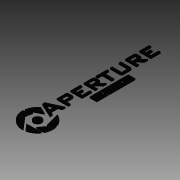
# Autodesk Inventor part: logo_full
Saved by Autodesk Inventor 2015 (Build 190159000, 159)
## iProperties
Created: 2014-10-14
Part Number: logo_full
Material: Generic
Document SubType Name: Modeling
Designer: Adam
Density: 1 g/cm^3
Appearance: Black
Author: Adam
Autodesk Inventor part; units mm, degrees
ref_plane "YZ Plane" through (0, 0, 0) normal (1, 0, 0) x (0, 1, 0)
ref_plane "XZ Plane" through (0, 0, 0) normal (0, 1, 0) x (-1, 0, 0)
ref_plane "XY Plane" through (0, 0, 0) normal (0, 0, 1) x (1, 0, 0)
sketch "Sketch1" plane through (0, 0, 0) normal (0, 1, 0) x (-1, 0, 0)
  line L0 (50, 0) -> (50, -199.1582) construction
  line L1 (50, -199.1582) -> (0, -199.1582) construction
  line L2 (0, -199.1582) -> (0, 0) construction
  line L3 (0, 0) -> (50, 0) construction
  line L4 (60, 0) -> (-10, 0) projected
  arc A0 (5.1979, -32.7466) -> (17.2152, -44.0591) centre (25, -23.75) ccw
  line L5 (11.7, -24) -> (5.1979, -32.7466)
  line L6 (11.7, -24) -> (17.2152, -44.0591)
  circle A1 centre (25, -23.75) radius 5.75
  arc A2 (5.6494, -13.8195) -> (4.2484, -30.2641) centre (25, -23.75) ccw
  line L7 (16.5428, -13.4822) -> (5.6494, -13.8195)
  line L8 (16.5428, -13.4822) -> (4.2484, -30.2641)
  arc A3 (20.7629, -2.4167) -> (7.0051, -11.5333) centre (25, -23.75) ccw
  line L9 (27.7937, -10.7443) -> (20.7629, -2.4167)
  line L10 (27.7937, -10.7443) -> (7.0051, -11.5333)
  arc A4 (39.0869, -7.1783) -> (23.3967, -2.0592) centre (25, -23.75) ccw
  line L11 (36.9278, -17.8609) -> (39.0869, -7.1783)
  line L12 (36.9278, -17.8609) -> (23.3967, -2.0592)
  arc A5 (46.7372, -24.4963) -> (41.0031, -9.0203) centre (25, -23.75) ccw
  line L13 (37.0241, -29.4397) -> (46.7372, -24.4963)
  line L14 (37.0241, -29.4397) -> (41.0031, -9.0203)
  arc A6 (37.9171, -41.2489) -> (46.4838, -27.1422) centre (25, -23.75) ccw
  line L15 (28.0098, -36.7074) -> (37.9171, -41.2489)
  line L16 (28.0098, -36.7074) -> (46.4838, -27.1422)
  line L17 (20.7257, -37.1631) -> (41.0031, -46.4582)
  line L18 (41.0031, -46.4582) -> (41.0031, -49.9857)
  line L19 (41.0031, -49.9857) -> (20.7257, -59.2364)
  line L20 (20.7257, -59.2364) -> (20.7257, -54.8042)
  line L21 (20.7257, -54.8042) -> (25.3171, -52.9285)
  line L22 (25.3171, -52.9285) -> (25.3171, -43.0274)
  line L23 (25.3171, -43.0274) -> (20.7257, -40.9227)
  line L24 (20.7257, -40.9227) -> (20.7257, -37.1631)
  line L25 (28.8648, -44.6536) -> (36.7381, -48.2627)
  line L26 (36.7381, -48.2627) -> (28.8648, -51.4791)
  line L27 (28.8648, -51.4791) -> (28.8648, -44.6536)
  line L28 (37.2257, -63.1991) -> (20.7257, -63.1991)
  line L29 (20.7257, -63.1991) -> (20.7257, -66.398)
  line L30 (27.2257, -66.398) -> (27.2257, -75.6295)
  line L31 (29.9757, -74.1295) -> (29.9757, -66.398)
  line L32 (37.2257, -63.1991) -> (37.2257, -75.6295)
  line L33 (34.4757, -74.1295) -> (34.4757, -66.398)
  arc A7 (34.7257, -78.1295) -> (37.2257, -75.6295) centre (34.7257, -75.6295) ccw
  arc A8 (27.2257, -75.6295) -> (29.7257, -78.1295) centre (29.7257, -75.6295) ccw
  line L34 (34.7257, -78.1295) -> (29.7257, -78.1295)
  line L35 (37.2257, -82.598) -> (20.7257, -82.598)
  line L36 (34.2257, -85.748) -> (34.2257, -96.6526)
  line L37 (34.2257, -96.6526) -> (37.2257, -96.6526)
  line L38 (37.2257, -96.6526) -> (37.2257, -82.598)
  line L39 (23.7257, -85.748) -> (23.7257, -96.6526)
  line L40 (23.7257, -96.6526) -> (20.7257, -96.6526)
  line L41 (20.7257, -96.6526) -> (20.7257, -82.598)
  arc A9 (33.4757, -75.1295) -> (34.4757, -74.1295) centre (33.4757, -74.1295) ccw
  arc A10 (29.9757, -74.1295) -> (30.9757, -75.1295) centre (30.9757, -74.1295) ccw
  line L42 (33.4757, -75.1295) -> (30.9757, -75.1295)
  line L43 (20.7257, -66.398) -> (27.2257, -66.398)
  line L44 (29.9757, -66.398) -> (34.4757, -66.398)
  line L45 (27.771, -85.748) -> (27.771, -92.1807)
  line L46 (27.771, -92.1807) -> (30.771, -92.1807)
  line L47 (30.771, -92.1807) -> (30.771, -85.748)
  line L48 (23.7257, -85.748) -> (27.771, -85.748)
  line L49 (30.771, -85.748) -> (34.2257, -85.748)
  line L50 (37.2257, -101.4125) -> (20.7257, -101.4125)
  line L51 (20.7257, -101.4125) -> (20.7257, -104.5625)
  arc A11 (33.4757, -113.1783) -> (34.4757, -112.1783) centre (33.4757, -112.1783) ccw
  arc A12 (29.9757, -112.1783) -> (30.9757, -113.1783) centre (30.9757, -112.1783) ccw
  line L52 (33.4757, -113.1783) -> (30.9757, -113.1783)
  line L53 (34.4757, -104.5625) -> (29.9757, -104.5625)
  line L54 (29.9757, -104.5625) -> (29.9757, -112.1783)
  line L55 (34.4757, -112.1783) -> (34.4757, -104.5625)
  arc A13 (34.7257, -116.1783) -> (37.2257, -113.6783) centre (34.7257, -113.6783) ccw
  arc A14 (27.2257, -113.6783) -> (29.7257, -116.1783) centre (29.7257, -113.6783) ccw
  line L56 (34.7257, -116.1783) -> (29.7257, -116.1783)
  line L57 (37.2257, -101.4125) -> (37.2257, -113.6783)
  line L58 (20.7257, -104.5625) -> (27.2257, -104.5625)
  line L59 (29.9757, -104.5625) -> (34.4757, -104.5625)
  line L60 (27.2257, -107.3837) -> (20.7257, -112.8855)
  line L61 (20.7257, -112.8855) -> (20.7257, -117.6583)
  line L62 (27.2257, -111.29) -> (20.7013, -117.6821)
  line L63 (37.2257, -101.4928) -> (37.2257, -101.4125)
  line L64 (37.2257, -113.6783) -> (37.2257, -113.1783)
  line L65 (37.2257, -101.4928) -> (37.2257, -101.4125)
  line L66 (37.2257, -118.6046) -> (34.2257, -118.6046)
  line L67 (34.2257, -134.6046) -> (37.2257, -134.6046)
  line L68 (37.2257, -134.6046) -> (37.2257, -118.6046)
  line L69 (34.2257, -124.8546) -> (20.7257, -124.8546)
  line L70 (20.7257, -124.8546) -> (20.7257, -128.3546)
  line L71 (20.7257, -128.3546) -> (34.2257, -128.3546)
  line L72 (34.2257, -118.6046) -> (34.2257, -124.8546)
  line L73 (34.2257, -128.3546) -> (34.2257, -134.6046)
  line L74 (37.2257, -126.6046) -> (20.7257, -126.6046) construction
  line L75 (27.2257, -104.5625) -> (27.2257, -107.3837)
  line L76 (27.2257, -111.29) -> (27.2257, -113.6783)
  line L77 (37.2257, -160.0956) -> (20.7257, -160.0956)
  line L78 (20.7257, -160.0956) -> (20.7257, -163.2456)
  arc A15 (33.4684, -171.8614) -> (34.4684, -170.8614) centre (33.4684, -170.8614) ccw
  arc A16 (29.9684, -170.8614) -> (30.9684, -171.8614) centre (30.9684, -170.8614) ccw
  line L79 (33.4684, -171.8614) -> (30.9684, -171.8614)
  line L80 (34.4684, -163.2456) -> (29.9684, -163.2456)
  line L81 (29.9684, -163.2456) -> (29.9684, -170.8614)
  line L82 (34.4684, -170.8614) -> (34.4684, -163.2456)
  arc A17 (34.7257, -174.8614) -> (37.2257, -172.3614) centre (34.7257, -172.3614) ccw
  arc A18 (27.2184, -172.3614) -> (29.7184, -174.8614) centre (29.7184, -172.3614) ccw
  line L83 (34.7257, -174.8614) -> (29.7184, -174.8614)
  line L84 (37.2257, -160.0956) -> (37.2257, -172.3614)
  line L85 (20.7257, -163.2456) -> (27.2184, -163.2456)
  line L86 (29.9684, -163.2456) -> (34.4684, -163.2456)
  line L87 (27.2184, -166.0668) -> (20.7257, -171.5759)
  line L88 (20.7257, -171.5759) -> (20.7257, -176.3487)
  line L89 (27.2184, -169.9731) -> (20.7137, -176.3605)
  line L90 (37.2257, -160.1464) -> (37.2257, -160.0956)
  line L91 (37.2257, -172.3614) -> (37.2257, -171.8614)
  line L92 (37.2257, -160.1464) -> (37.2257, -160.0956)
  line L93 (27.2184, -163.2456) -> (27.2184, -166.0668)
  line L94 (27.2184, -169.9731) -> (27.2184, -172.3614)
  line L95 (37.2257, -180.2989) -> (20.7257, -180.2989)
  line L96 (34.2257, -183.4489) -> (34.2257, -194.3535)
  line L97 (34.2257, -194.3535) -> (37.2257, -194.3535)
  line L98 (37.2257, -194.3535) -> (37.2257, -180.2989)
  line L99 (23.7257, -183.4489) -> (23.7257, -194.3535)
  line L100 (23.7257, -194.3535) -> (20.7257, -194.3535)
  line L101 (20.7257, -194.3535) -> (20.7257, -180.2989)
  line L102 (27.771, -183.4489) -> (27.771, -189.8816)
  line L103 (27.771, -189.8816) -> (30.771, -189.8816)
  line L104 (30.771, -189.8816) -> (30.771, -183.4489)
  line L105 (23.7257, -183.4489) -> (27.771, -183.4489)
  line L106 (30.771, -183.4489) -> (34.2257, -183.4489)
  line L107 (37.2257, -138.6629) -> (23.4227, -138.6629)
  line L108 (23.7257, -141.8629) -> (37.2257, -141.8629)
  line L109 (37.2257, -141.8629) -> (37.2257, -138.6629)
  line L110 (37.2257, -150.938) -> (23.7257, -150.938)
  line L111 (23.4227, -154.138) -> (37.2257, -154.138)
  line L112 (37.2257, -154.138) -> (37.2257, -150.938)
  line L113 (23.7257, -150.938) -> (23.7257, -141.8629)
  arc A19 (20.7257, -151.4409) -> (23.4227, -154.138) centre (23.4227, -151.4409) ccw
  arc A20 (23.4227, -138.6629) -> (20.7257, -141.36) centre (23.4227, -141.36) ccw
  line L114 (20.7257, -141.36) -> (20.7257, -151.4409)
  line L115 (16.0446, -88.9644) -> (6.0602, -88.9644)
  line L116 (6.0602, -88.9644) -> (6.0602, -143.5469)
  line L117 (6.0602, -143.5469) -> (16.0446, -143.5469)
  line L118 (16.0446, -143.5469) -> (16.0446, -88.9644)
  dimension "d9" = 50
  dimension "d17" = 52
  dimension "d24" = 20.8035
  dimension "d25" = 21.75
  dimension "d26" = 11.7
  dimension "d28" = 24
  dimension "d54" = 25
  dimension "d56" = 23.75
  dimension "d57" = 11.5
  dimension "d64" = 258
  dimension "d252" = 2.5
  dimension "d255" = 16.5
  dimension "d258" = 6.5
  dimension "d259" = 2.75
  dimension "d260" = 2.75
  dimension "d261" = 1
  dimension "d262" = 3.15
  dimension "d265" = 16.2
  dimension "d271" = 3
  dimension "d273" = 3
  dimension "d280" = 3
  dimension "d282" = 3
  dimension "d283" = 3
  dimension "d284" = 3.15
  dimension "d295" = 3
  dimension "d296" = 3.5
  dimension "d297" = 16
  dimension "d305" = 3
  dimension "d306" = 3.15
  dimension "d312" = 2.75
  dimension "d313" = 2.8212
  dimension "d320" = 16.5
  dimension "d321" = 3.15
  dimension "d322" = 3
  dimension "d323" = 3
  dimension "d324" = 3
  dimension "d351" = 3.2
  dimension "d352" = 3.2
  dimension "d353" = 3
  constraints: 228 end point, 45 parallel, 40 point on circle, 32 collinear, 30 tangent, 21 centre point, 16 horizontal, 10 point on line, 10 vertical, 9 perpendicular, 7 equal radius, 3 coincident, 2 midpoint, 1 vertical alignment, 37 other
  measures "d9" distance of L0.end L1.end
  measures "d17" angle of L5 L6
  measures "d24" distance of L5.start L6.end
  measures "d25" radius of A0
  measures "d26" distance from line of L2 L5.start
  measures "d28" distance from line of L3 L5.start
  measures "d54" distance from line of L2 A1.centre
  measures "d56" distance from line of L3 A1.centre
  measures "d57" diameter of A1
  measures "d252" radius of A7
  measures "d255" distance of L35.start L35.end
  measures "d258" distance between parallel lines of L41 L30
  measures "d259" distance between parallel lines of L31 L30
  measures "d260" distance between parallel lines of L32 L33
  measures "d261" radius of A9
  measures "d262" distance between parallel lines of L35 L49
  measures "d265" distance between parallel lines of L43 L35
  measures "d271" distance between parallel lines of L34 L42
  measures "d273" distance between parallel lines of L56 L52
  measures "d280" distance between parallel lines of L36 L38
  measures "d282" distance between parallel lines of L45 L47
  measures "d283" distance between parallel lines of L41 L39
  measures "d284" distance between parallel lines of L50 L53
  measures "d295" distance between parallel lines of L72 L68
  measures "d296" distance between parallel lines of L71 L69
  measures "d297" distance of L67.end L66.start
  measures "d305" distance between parallel lines of L83 L79
  measures "d306" distance between parallel lines of L77 L80
  measures "d312" distance between parallel lines of L81 L93
  measures "d313" distance of L93.start L93.end
  measures "d320" distance of L95.start L95.end
  measures "d321" distance between parallel lines of L95 L106
  measures "d322" distance between parallel lines of L96 L98
  measures "d323" distance between parallel lines of L102 L104
  measures "d324" distance between parallel lines of L101 L99
  measures "d351" distance of L111.end L110.start
  measures "d352" distance of L108.end L107.start
  measures "d353" distance between parallel lines of L114 L113
extrude "Extrusion1" add sketch "Sketch1" along normal blind 2
sketch "Sketch2" plane through (0, 2, 0) normal (0, 1, 0) x (1, 0, 0)
  line L0 (-14.0025, 91.7025) -> (-14.0025, 151.1401) construction
  line L1 (-14.0025, 151.1401) -> (-8.0025, 151.1401) construction
  line L2 (-8.0025, 151.1401) -> (-8.0025, 91.7025) construction
  line L3 (-8.0025, 91.7025) -> (-14.0025, 91.7025) construction
  line L4 (-8.0025, 126.4644) -> (-14.0025, 126.4644)
  line L5 (-14.0025, 126.4644) -> (-14.0025, 127.5644)
  line L6 (-14.0025, 127.5644) -> (-10.7116, 129.4644)
  line L7 (-10.7116, 129.4644) -> (-14.0025, 131.3644)
  line L8 (-14.0025, 131.3644) -> (-14.0025, 132.4644)
  line L9 (-14.0025, 132.4644) -> (-8.0025, 132.4644)
  line L10 (-8.0025, 132.4644) -> (-8.0025, 131.3644)
  line L11 (-8.0025, 131.3644) -> (-12.0025, 131.3644)
  line L12 (-12.0025, 131.3644) -> (-8.7116, 129.4644)
  line L13 (-8.7116, 129.4644) -> (-12.0025, 127.5644)
  line L14 (-12.0025, 127.5644) -> (-8.0025, 127.5644)
  line L15 (-8.0025, 126.4644) -> (-8.0025, 127.5644)
  line L16 (-6.0602, 88.9644) -> (-6.0602, 143.5469) projected
  line L17 (-16.0446, 88.9644) -> (-6.0602, 88.9644) projected
  line L18 (-12.7651, 96.9555) -> (-12.7651, 94.1247)
  line L19 (-12.7651, 94.1247) -> (-11.7554, 94.1247)
  line L20 (-11.7554, 94.1247) -> (-11.7554, 96.9263)
  spline S0 degree 2 poles (-11.7554, 96.9263) (-11.7554, 97.6675) (-11.1017, 98.2103) (-10.2788, 98.2103) knots 0 0 0 1 2 2 2
  line L21 (-10.2788, 98.2103) -> (-9.485, 98.2103)
  spline S1 degree 2 poles (-9.485, 98.2103) (-8.6562, 98.2103) (-8.0025, 97.6675) (-8.0025, 96.9263) knots 0 0 0 1 2 2 2
  line L22 (-8.0025, 96.9263) -> (-8.0025, 94.0372)
  spline S2 degree 2 poles (-8.0025, 94.0372) (-8.0025, 93.2901) (-8.6504, 92.7473) (-9.485, 92.7473) knots 0 0 0 1 2 2 2
  line L23 (-9.485, 92.7473) -> (-9.7243, 92.7473)
  line L24 (-9.7243, 92.7473) -> (-10.0044, 93.9438)
  line L25 (-10.0044, 93.9438) -> (-9.3157, 93.9438)
  line L26 (-9.3157, 93.9438) -> (-9.3157, 97.0138)
  line L27 (-9.3157, 97.0138) -> (-10.4072, 97.0138)
  line L28 (-10.4072, 97.0138) -> (-10.4072, 94.2181)
  spline S3 degree 2 poles (-10.4072, 94.2181) (-10.4072, 93.4769) (-11.0609, 92.9399) (-11.8897, 92.9399) knots 0 0 0 1 2 2 2
  line L29 (-11.8897, 92.9399) -> (-12.5258, 92.9399)
  spline S4 degree 2 poles (-12.5258, 92.9399) (-13.3546, 92.9399) (-14.0025, 93.4769) (-14.0025, 94.2181) knots 0 0 0 1 2 2 2
  line L30 (-14.0025, 94.2181) -> (-14.0025, 96.8737)
  spline S5 degree 2 poles (-14.0025, 96.8737) (-14.0025, 97.5858) (-13.3721, 98.1519) (-12.6251, 98.1519) knots 0 0 0 1 2 2 2
  line L31 (-12.6251, 98.1519) -> (-12.4149, 98.1519)
  line L32 (-12.4149, 98.1519) -> (-12.1114, 96.9555)
  line L33 (-12.1114, 96.9555) -> (-12.7651, 96.9555)
  line L34 (-8.0025, 101.6889) -> (-10.664, 101.6889)
  line L35 (-10.664, 101.6889) -> (-14.0025, 99.2609)
  line L36 (-14.0025, 99.2609) -> (-14.0025, 100.8893)
  line L37 (-14.0025, 100.8893) -> (-11.7904, 102.436)
  line L38 (-11.7904, 102.436) -> (-14.0025, 103.9827)
  line L39 (-14.0025, 103.9827) -> (-14.0025, 105.4418)
  line L40 (-14.0025, 105.4418) -> (-10.699, 103.0197)
  line L41 (-10.699, 103.0197) -> (-8.0025, 103.0197)
  line L42 (-8.0025, 103.0197) -> (-8.0025, 101.6889)
  line L43 (-12.7651, 110.6597) -> (-12.7651, 107.829)
  line L44 (-12.7651, 107.829) -> (-11.7554, 107.829)
  line L45 (-11.7554, 107.829) -> (-11.7554, 110.6305)
  spline S6 degree 2 poles (-11.7554, 110.6305) (-11.7554, 111.3718) (-11.1017, 111.9146) (-10.2788, 111.9146) knots 0 0 0 1 2 2 2
  line L46 (-10.2788, 111.9146) -> (-9.485, 111.9146)
  spline S7 degree 2 poles (-9.485, 111.9146) (-8.6562, 111.9146) (-8.0025, 111.3718) (-8.0025, 110.6305) knots 0 0 0 1 2 2 2
  line L47 (-8.0025, 110.6305) -> (-8.0025, 107.7414)
  spline S8 degree 2 poles (-8.0025, 107.7414) (-8.0025, 106.9944) (-8.6504, 106.4516) (-9.485, 106.4516) knots 0 0 0 1 2 2 2
  line L48 (-9.485, 106.4516) -> (-9.7243, 106.4516)
  line L49 (-9.7243, 106.4516) -> (-10.0044, 107.6481)
  line L50 (-10.0044, 107.6481) -> (-9.3157, 107.6481)
  line L51 (-9.3157, 107.6481) -> (-9.3157, 110.7181)
  line L52 (-9.3157, 110.7181) -> (-10.4072, 110.7181)
  line L53 (-10.4072, 110.7181) -> (-10.4072, 107.9224)
  spline S9 degree 2 poles (-10.4072, 107.9224) (-10.4072, 107.1811) (-11.0609, 106.6442) (-11.8897, 106.6442) knots 0 0 0 1 2 2 2
  line L54 (-11.8897, 106.6442) -> (-12.5258, 106.6442)
  spline S10 degree 2 poles (-12.5258, 106.6442) (-13.3546, 106.6442) (-14.0025, 107.1811) (-14.0025, 107.9224) knots 0 0 0 1 2 2 2
  line L55 (-14.0025, 107.9224) -> (-14.0025, 110.578)
  spline S11 degree 2 poles (-14.0025, 110.578) (-14.0025, 111.2901) (-13.3721, 111.8562) (-12.6251, 111.8562) knots 0 0 0 1 2 2 2
  line L56 (-12.6251, 111.8562) -> (-12.4149, 111.8562)
  line L57 (-12.4149, 111.8562) -> (-12.1114, 110.6597)
  line L58 (-12.1114, 110.6597) -> (-12.7651, 110.6597)
  line L59 (-12.7418, 116.5021) -> (-8.0025, 116.5021)
  line L60 (-8.0025, 116.5021) -> (-8.0025, 115.1772)
  line L61 (-8.0025, 115.1772) -> (-12.7418, 115.1772)
  line L62 (-12.7418, 115.1772) -> (-12.7418, 113.0294)
  line L63 (-12.7418, 113.0294) -> (-14.0025, 113.0294)
  line L64 (-14.0025, 113.0294) -> (-14.0025, 118.6558)
  line L65 (-14.0025, 118.6558) -> (-12.7418, 118.6558)
  line L66 (-12.7418, 118.6558) -> (-12.7418, 116.5021)
  line L67 (-8.0025, 119.8757) -> (-14.0025, 119.8757)
  line L68 (-14.0025, 119.8757) -> (-14.0025, 124.901)
  line L69 (-14.0025, 124.901) -> (-12.7943, 124.901)
  line L70 (-12.7943, 124.901) -> (-12.7943, 121.2006)
  line L71 (-12.7943, 121.2006) -> (-11.7262, 121.2006)
  line L72 (-11.7262, 121.2006) -> (-11.7262, 123.3601)
  line L73 (-11.7262, 123.3601) -> (-10.5181, 123.3601)
  line L74 (-10.5181, 123.3601) -> (-10.5181, 121.2006)
  line L75 (-10.5181, 121.2006) -> (-9.3157, 121.2006)
  line L76 (-9.3157, 121.2006) -> (-9.3157, 124.9477)
  line L77 (-9.3157, 124.9477) -> (-8.0025, 124.9477)
  line L78 (-8.0025, 124.9477) -> (-8.0025, 119.8757)
  line L79 (-12.7651, 138.0858) -> (-12.7651, 135.2551)
  line L80 (-12.7651, 135.2551) -> (-11.7554, 135.2551)
  line L81 (-11.7554, 135.2551) -> (-11.7554, 138.0566)
  spline S12 degree 2 poles (-11.7554, 138.0566) (-11.7554, 138.7979) (-11.1017, 139.3407) (-10.2788, 139.3407) knots 0 0 0 1 2 2 2
  line L82 (-10.2788, 139.3407) -> (-9.485, 139.3407)
  spline S13 degree 2 poles (-9.485, 139.3407) (-8.6562, 139.3407) (-8.0025, 138.7979) (-8.0025, 138.0566) knots 0 0 0 1 2 2 2
  line L83 (-8.0025, 138.0566) -> (-8.0025, 135.1675)
  spline S14 degree 2 poles (-8.0025, 135.1675) (-8.0025, 134.4204) (-8.6504, 133.8776) (-9.485, 133.8776) knots 0 0 0 1 2 2 2
  line L84 (-9.485, 133.8776) -> (-9.7243, 133.8776)
  line L85 (-9.7243, 133.8776) -> (-10.0044, 135.0741)
  line L86 (-10.0044, 135.0741) -> (-9.3157, 135.0741)
  line L87 (-9.3157, 135.0741) -> (-9.3157, 138.1442)
  line L88 (-9.3157, 138.1442) -> (-10.4072, 138.1442)
  line L89 (-10.4072, 138.1442) -> (-10.4072, 135.3484)
  spline S15 degree 2 poles (-10.4072, 135.3484) (-10.4072, 134.6072) (-11.0609, 134.0702) (-11.8897, 134.0702) knots 0 0 0 1 2 2 2
  line L90 (-11.8897, 134.0702) -> (-12.5258, 134.0702)
  spline S16 degree 2 poles (-12.5258, 134.0702) (-13.3546, 134.0702) (-14.0025, 134.6072) (-14.0025, 135.3484) knots 0 0 0 1 2 2 2
  line L91 (-14.0025, 135.3484) -> (-14.0025, 138.0041)
  spline S17 degree 2 poles (-14.0025, 138.0041) (-14.0025, 138.7162) (-13.3721, 139.2823) (-12.6251, 139.2823) knots 0 0 0 1 2 2 2
  line L92 (-12.6251, 139.2823) -> (-12.4149, 139.2823)
  line L93 (-12.4149, 139.2823) -> (-12.1114, 138.0858)
  line L94 (-12.1114, 138.0858) -> (-12.7651, 138.0858)
  point P0 (0, 0)
  dimension "d383" = 1.1
  dimension "d384" = 1.9423
  dimension "d385" = 2.7382
  dimension "d386" = 30
  dimension "d387" = 1.1
  dimension "d388" = 1
  dimension "d389" = 1
  dimension "d390" = 6
  dimension "d391" = 6
  dimension "d392" = 37.5
  constraints: 24 end point, 8 point on line, 2 horizontal, 2 horizontal alignment, 2 parallel, 2 perpendicular, 1 collinear, 1 vertical alignment, 2 other
  measures "d383" distance of L4.start L14.end
  measures "d384" distance between parallel lines of L16 L2
  measures "d385" distance between parallel lines of L17 L3
  measures "d386" angle of L14 L13
  measures "d387" distance between parallel lines of L11 L9
  measures "d388" distance between parallel lines of L12 L7
  measures "d389" distance between parallel lines of L13 L6
  measures "d390" distance between parallel lines of L9 L4
  measures "d391" distance between parallel lines of L2 L0
  measures "d392" distance between parallel lines of L17 L4
extrude "Extrusion2" cut sketch "Sketch2" against normal through all
equation "\"d273\" = d271"
body "Solid1"
